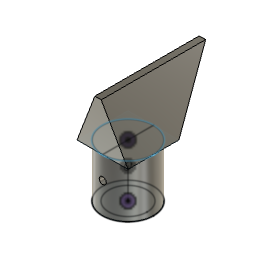
car_scraper_2 (Autodesk Fusion 360 design; units mm, degrees)
Autodesk Fusion 360 part; units mm, degrees
note: some values were not read from the file. Set by a fixed rule: which face or edge a step refers to.
sketch "Sketch1" plane through (0, 0, 0) normal (0, 0, 1) x (1, 0, 0)
  circle A0 centre (0, 0) radius 9.75
  circle A1 centre (0, 0) radius 13
  dimension "d1" = 19.5
  dimension "d2" = 26
  constraint coincident A0.centre A1.centre
  measures "d1" diameter of A0
  measures "d2" diameter of A1
extrude "Extrude1" add sketch "Sketch1" along normal blind 25 makes body 1
sketch "Sketch2" plane through (0, 0, 0) normal (0, 1, 0) x (1, 0, 0)
  line L0 (0, 0) -> (0, -15.5)
  circle A0 centre (0, -15.5) radius 1.75
  dimension "d5" = 15.5
  dimension "d6" = 3.5
  constraint coincident L0.start origin
  constraint vertical L0
  constraint coincident L0.end A0.centre
  measures "d5" distance of L0.start L0.end
  measures "d6" diameter of A0
extrude "Extrude2" cut sketch "Sketch2" against normal blind 100 bodies 1
sketch "Sketch3" plane through (0, 0, 25) normal (0, 0, 1) x (-1, 0, 0)
  circle A0 centre (0, 0) radius 9.75
  circle A1 centre (0, 0) radius 13
  circle A2 centre (0, 0) radius 13
  constraint coincident A0.centre A1.centre
extrude "Extrude3" add sketch "Sketch3" along normal blind 35 contours A0 | A1 A2 bodies 1
sketch "Sketch4" plane through (0, 0, 0) normal (0, 1, 0) x (1, 0, 0)
  line L0 (0, -60) -> (-13, -25)
  line L1 (-13, -25) -> (13, -25)
  line L2 (13, -25) -> (0, -60)
  line L3 (-13, -25) -> (13, -25)
  line L4 (13, -25) -> (13, -60)
  line L5 (13, -60) -> (-13, -60)
  line L6 (-13, -60) -> (-13, -25)
  constraint horizontal L1
  constraint horizontal L3
  constraint vertical L4
  constraint horizontal L5
  constraint vertical L6
extrude "Extrude4" cut sketch "Sketch4" along normal blind 100 contours L0 L5 L6 | L2 L4 L5 bodies 1
extrude "Extrude5" cut 2 faces at (-8.6667, 0, 48.3333) (8.6667, 0, 48.3333) along direction (0, -1, 0) blind 100 on bodies 1 bodies 1
sketch "Sketch5" plane through (0, 0, 0) normal (1, 0, 0) x (0, 1, 0)
  line L0 (0, 25) -> (35, 85.6218)
  line L1 (0, 25) -> (50, 25) construction
  line L2 (0, 25) -> (-35, 85.6218)
  line L3 (0, 25) -> (50, 25) construction
  line L4 (-35, 85.6218) -> (35, 85.6218)
  line L5 (-13, 60) -> (-13, 47.5167)
  line L6 (13, 60) -> (13, 47.5167)
  line L7 (-13, 60) -> (13, 60)
  dimension "d17" = 60
  dimension "d18" = 70
  dimension "d19" = 120
  dimension "d20" = 70
  constraint horizontal L1
  constraint horizontal L3
  constraint coincident L2 L5.end
  constraint vertical L5
  constraint coincident L0 L6.end
  constraint parallel L5 L6
  constraint perpendicular L6 L7
  measures "d17" angle of L0 L1
  measures "d18" distance of L0.start L0.end
  measures "d19" angle of L2 L3
  measures "d20" distance of L0.start L2.end
extrude "Extrude6" add sketch "Sketch5" along normal blind 2.5 separate body contours L0 L2 L4 L5 L6 L7 makes body 2
extrude "Extrude7" add 1 faces at (0, 4.3333, 77.0812) along direction (-1, 0, 0) blind 2.5 on bodies 2 bodies 1 2
extrude "Extrude8" cut 1 faces at (-1.6667, 0, 60) along direction (0, 0, -1) blind 10 on bodies 1 bodies 1
extrude "Extrude9" add 1 faces at (-1.6667, 0, 60) along direction (0, 0, -1) blind 10 on bodies 1 bodies 1
extrude "Extrude10" cut 1 faces at (1.6667, 0, 60) along direction (0, 0, -1) blind 10 on bodies 1 bodies 1
extrude "Extrude11" add 1 faces at (1.6667, 0, 60) along direction (0, 0, -1) blind 10 on bodies 1 bodies 1
extrude "Extrude12" cut 1 faces at (1.6667, -13, 49.1722) along direction (0, 1, 0) blind 26 on bodies 1 bodies 1
extrude "Extrude13" add 1 faces at (1.6667, -13, 49.1722) along direction (0, 1, 0) blind 26 on bodies 1 bodies 1
fillet "Fillet1" radius 1 2 edges at (0, -35, 85.6218) (0, 35, 85.6218) on bodies 1
sketch "Sketch7" plane through (0, 0, 0) normal (0, 1, 0) x (1, 0, 0)
  line L0 (-1.5, -86) -> (3, -86)
  line L1 (3, -86) -> (3, -81.5)
  line L2 (3, -81.5) -> (-1.5, -86)
  constraint horizontal L0
  constraint perpendicular L0 L1
extrude "Extrude14" cut sketch "Sketch7" along normal blind 100 bodies 1
extrude "Extrude15" cut 1 faces at (1.2927, 0, 84.4145) along direction (0, -1, 0) blind 100 on bodies 1 bodies 1
fillet "Fillet2" radius 1 6 edges at (2.5, 0, 82) (1.4391, -33.5215, 83.0609) (-0.6218, -34.134, 85.1218) (-1.1218, 0, 85.6218) (-0.6218, 34.134, 85.1218) (1.4391, 33.5215, 83.0609) on bodies 1
sketch "Sketch8" plane through (0, 0, 0) normal (1, 0, 0) x (0, 1, 0)
  line L0 (0, 0) -> (0, 15.5)
  circle A0 centre (0, 15.5) radius 1.75
  dimension "d45" = 15.5
  dimension "d46" = 3.5
  constraint coincident L0.start origin
  constraint vertical L0
  constraint coincident L0.end A0.centre
  measures "d45" distance of L0.start L0.end
  measures "d46" diameter of A0
extrude "Extrude16" cut sketch "Sketch8" against normal blind 100 bodies 1
sketch "Sketch9" plane through (0, 0, 85.6218) normal (0, 0, 1) x (-1, 0, 0)
  line L0 (1.536, 33.2679) -> (1.536, -33.2679)
  line L1 (1.536, -33.2679) -> (2.5, -33.2679)
  line L2 (2.5, -33.2679) -> (2.5, 33.2679)
  line L3 (2.5, 33.2679) -> (1.536, 33.2679)
  line L4 (26.6391, -37.0169) -> (-34.8106, -37.0169)
  line L5 (-34.8106, -37.0169) -> (-34.8106, 39.1415)
  line L6 (-34.8106, 39.1415) -> (26.6391, 39.1415)
  line L7 (26.6391, 39.1415) -> (26.6391, -37.0169)
  constraint horizontal L4
  constraint vertical L5
  constraint horizontal L6
  constraint vertical L7
extrude "Extrude17" cut sketch "Sketch9" against normal blind 61 contours L0 L1 L2 L3 | L4 L5 L6 L7 bodies 1
extrude "Extrude18" add 1 faces at (11.8683, 0.6458, 24.6218) along direction (0, 0, 1) blind 2 on bodies 1 bodies 1
extrude "Extrude19" add sketch "Sketch1" along normal blind 27 contours A0 bodies 1
extrude "Extrude20" add 1 faces at (11.8683, 0.6458, 26.6218) along direction (0, 0, 1) blind 0.4 on bodies 1 bodies 1
extrude "Extrude21" cut sketch "Sketch9" against normal blind 58.7 contours L0 L1 L2 L3 | L4 L5 L6 L7 bodies 1
sketch "Sketch10" plane through (0, 0, 0) normal (1, 0, 0) x (0, 1, 0)
  line L0 (13, 27) -> (26.6808, 64.5877)
  line L1 (13, 27) -> (53, 27) construction
  line L2 (-13, 27) -> (-26.6808, 64.5877)
  line L3 (-13, 27) -> (27, 27) construction
  line L4 (26.6808, 64.5877) -> (-26.6808, 64.5877)
  line L5 (13, 27) -> (-13, 27)
  dimension "d59" = 70
  dimension "d60" = 40
  dimension "d61" = 110
  dimension "d62" = 40
  constraint horizontal L1
  constraint horizontal L3
  constraint horizontal L4
  measures "d59" angle of L0 L1
  measures "d60" distance of L0.start L0.end
  measures "d61" angle of L2 L3
  measures "d62" distance of L2.start L2.end
extrude "Extrude22" add sketch "Sketch10" along normal blind 13 separate body makes body 3
extrude "Extrude23" add 1 faces at (0, -4.3333, 52.0585) along direction (-1, 0, 0) blind 13 on bodies 3 bodies 3
sketch "Sketch11" plane through (0, 0, 27) normal (0, 0, -1) x (1, 0, 0)
  line L0 (-13, -13) -> (13, -13)
  line L1 (13, -13) -> (13, 13)
  line L2 (13, 13) -> (-13, 13)
  line L3 (-13, 13) -> (-13, -13)
  line L4 (0, 13) -> (0, -13)
  circle A0 centre (0, 0) radius 13.1529
  circle A1 centre (0, 0) radius 13
  constraint midpoint L2 L4.start
  constraint midpoint L0 L4.end
  constraint coincident A0.centre A1.centre
  constraint concentric A0 A1
  constraint coincident L4.start A1
sketch "Sketch12" plane through (0, 0, 0) normal (0, 1, 0) x (1, 0, 0)
  line L0 (-13, -27) -> (13, -27)
  line L1 (13, -27) -> (13, -70)
  line L2 (13, -70) -> (-13, -27)
  line L3 (-13, -27) -> (-13, -70)
  line L4 (-13, -70) -> (13, -70)
  constraint horizontal L0
  constraint perpendicular L0 L1
  constraint perpendicular L0 L3
  constraint perpendicular L1 L4
extrude "Extrude24" cut sketch "Sketch12" against normal blind 100 contours L2 L3 L4 bodies 3
extrude "Extrude25" cut sketch "Sketch12" along normal blind 100 contours L2 L3 L4 bodies 3
extrude "Extrude26" cut sketch "Sketch1" along normal blind 26 contours A0 bodies 1
